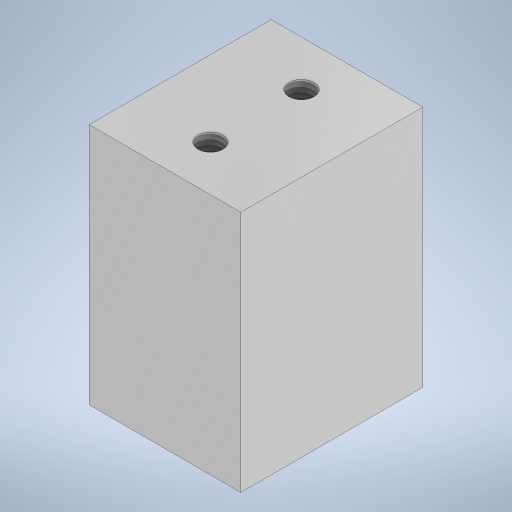
# Autodesk Inventor part: Suporte da probe
Saved by Autodesk Inventor 2023 (Build 270158000, 158)
## iProperties
Created: 2023-03-31
Part Number: Suporte da probe
Material: Alumínio 6061
Document SubType Name: Sheet Metal
Designer: Mateus PC
Density: 2.7 g/cm^3
Sheet Metal Rule: Default_mm
Appearance: Usinado - Alumínio
Mass: 44.6499 g
Surface Area: 56.5011 cm^2
Volume: 16.537 cm^3
Author: Mateus PC
Autodesk Inventor part; units mm, degrees
ref_plane "YZ Plane" through (0, 0, 0) normal (1, 0, 0) x (0, 1, 0)
ref_plane "XZ Plane" through (0, 0, 0) normal (0, 1, 0) x (-1, 0, 0)
ref_plane "XY Plane" through (0, 0, 0) normal (0, 0, 1) x (1, 0, 0)
sketch "Esboço1" plane through (0, 0, 0) normal (0, 1, 0) x (-1, 0, 0)
  line L0 (0, 0) -> (25, 0)
  line L1 (25, 0) -> (25, -30)
  line L2 (25, -30) -> (0, -30)
  line L3 (0, -30) -> (0, 0)
  dimension "d0" = 25
  dimension "d1" = 30
  constraints: 8 end point, 2 parallel, 1 horizontal, 1 perpendicular
  measures "d0" distance of L1.end L2.end
  measures "d1" distance of L0.end L1.end
extrude "Extrusão1" add sketch "Esboço1" along normal blind 20
sketch "Esboço2" plane through (0, 20, 0) normal (0, 1, 0) x (1, 0, 0)
  line L0 (0, 30) -> (-25, 30) projected
  line L1 (-25, 30) -> (-25, 0) projected
  line L2 (-25, 0) -> (0, 0) projected
  point P0 (-12.5, 7.5)
  point P1 (-12.5, 22.5)
  point P2 (-12.5, 30)
  point P3 (-12.5, 0)
  dimension "d4" = 25
  dimension "d5" = 12.5
  dimension "d6" = 12.5
  dimension "d31" = 7.5
  dimension "d32" = 7.5
  constraints: 2 midpoint
  measures "d4" distance of L0.start L0.end
  measures "d5" distance from line of point (-12.5, 22.5) L1
  measures "d6" distance from line of L1 point (-12.5, 7.5)
  measures "d31" distance from line of point (-12.5, 22.5) L0
  measures "d32" distance from line of L2 point (-12.5, 7.5)
hole "Furo1" at (-12.5, 20, -7.5) at (-12.5, 20, -22.5) direction (0, -1, 0) diameter 4.134 depth 14.2 tip angle 118 thread size "M5x0.8" class "6H" standard "ISO Metric profile"
sketch "Esboço3" plane through (0, 0, 0) normal (0, -1, 0) x (1, 0, 0)
  circle A0 centre (-12.5, -15) radius 7.5 construction
  line L0 (0, 0) -> (0, -30) projected
  line L1 (0, -30) -> (-25, -30) projected
  line L2 (-25, -30) -> (-25, 0) projected
  line L3 (0, -30) -> (-25, -30) projected
  line L4 (0, 0) -> (0, -30) projected
  line L5 (-25, 0) -> (0, 0) projected
  dimension "d16" = 25
  dimension "d17" = 30
  dimension "d18" = 12.5
  dimension "d19" = 15
  dimension "d21" = 15
  constraints: 1 centre point
  measures "d16" distance of L0.end L1.end
  measures "d17" distance of L0.start L0.end
  measures "d18" distance from line of L0 A0.centre
  measures "d19" distance from line of L1 A0.centre
  measures "d21" diameter of A0
extrude "Extrusão2" add sketch "Esboço3" along normal blind 20
sketch "Esboço5" plane through (-12.5, -20, -15) normal (0, -1, 0) x (1, 0, 0)
  circle A0 centre (0, 0) radius 7.5 projected
  point P0 (12.5, 15)
  constraints: 1 coincident
hole "Furo3" at (-12.5, -20, -15) direction (0, 1, 0) diameter 8.376 depth 20 tip angle 118 thread size "M10x1.5" class "6H" standard "ISO Metric profile"
equation "\"d6\" = d5"
equation "\"d32\" = d31"
equation "\"d18\" = 0.5 * d16"
equation "\"d19\" = 0.5 * d17"
equation "\"Raio_vergadura\" = Espessura"
equation "\"Largura_alívio_de_vergadura\" = Espessura"
equation "\"Profundidade_alívio_de_vergadura\" = 0.5 * Espessura"
equation "\"Tamanho_alívio_de_dobra\" = 4 * Espessura"
equation "\"Remanescente_mínimo\" = 2 * Espessura"
equation "\"Raiodetransição\" = Raio_vergadura"
equation "\"Tamanho_de_raio_de_Jacobi\" = Raio_vergadura"
equation "\"TamanhoFolga\" = Espessura"
equation "\"Espessura\" = 0.5"
